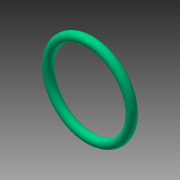
# Autodesk Inventor part: o_ring_4.29_0.5XXX
Saved by Autodesk Inventor 2015 (Build 190159000, 159)
## iProperties
Created: 2015-01-11
Part Number: o_ring_4.29_0.5XXX
Material: Generic
Document SubType Name: Modeling
Designer: ice
Density: 1 g/cm^3
Appearance: Default
Mass: 0.00295471 g
Surface Area: 0.236377 cm^2
Volume: 0.00295471 cm^3
Author: ice
Autodesk Inventor part; units mm, degrees
ref_plane "YZ Plane" through (0, 0, 0) normal (1, 0, 0) x (0, 1, 0)
ref_plane "XZ Plane" through (0, 0, 0) normal (0, 1, 0) x (-1, 0, 0)
ref_plane "XY Plane" through (0, 0, 0) normal (0, 0, 1) x (1, 0, 0)
sketch "Sketch1" plane through (0, 0, 0) normal (0, 0, 1) x (1, 0, 0)
  line L0 (0, -2.136) -> (0, 2.2442)
  line L1 (0, 0) -> (2.145, 0) construction
  circle A0 centre (2.395, 0) radius 0.25
  line L2 (2.145, 0) -> (2.145, 0.4659)
  dimension "d6" = 2.145
  constraints: 6 end point, 2 point on circle, 2 vertical, 1 centre point, 1 horizontal, 1 tangent
  measures "d6" distance between parallel lines of L0 L2
revolve "Revolution1" add sketch "Sketch1" angle 360 about axis through (0, -2.136, 0) along (0, 1, 0)
body "Solid1"
